Autodesk Fusion 360 part; units mm, degrees
note: some values were not read from the file. Chosen so that the rebuilt part matches the saved one: which face or edge a step refers to.
(part 2 of 2)
extrude "Extrusion14" cut sketch "Skizze12" against normal blind 11 contours L16 L18 L19 L481 L482 | L16 L475 L476 L477 | L18 L414 L418 | L16 L469 L470 L471 | L13 L408 L409 L410 L411 L412 L413 | L16 L463 L464 L465 | L16 L457 L458 L459 | L16 L451 L452 L453 | L14 L342 L343 L344 L345 L346 L347 | L16 L445 L446 L447 | L14 L276 L280 | L16 L439 L440 L441 | L14 L270 L271 L272 L273 L274 L275 | L16 L433 L434 L435 | L14 L204 L208 | L16 L427 L428 L429 | L14 L198 L199 L200 L201 L202 L203 | L16 L17 L20 L21 L422 L423 | L14 L132 L136 | L14 L15 L126 L127 L128 L129 L130 L131 | L17 L364 L365 | L15 L366 L367 L368 L369 L370 L371 | L15 L124 L125 | L15 L186 L187 L188 L189 L190 L191 | L15 L306 L307 L308 L309 L310 L311 | L15 L184 L185 | L15 L244 L245 | L15 L246 L247 L248 L249 L250 L251 | L24 L25 L26 L27 L28 L29 | L192 L193 L194 L195 L196 L197 | L252 L253 L254 L255 L256 L257 | L258 L259 L260 L261 L262 L263 | L264 L265 L266 L267 L268 L269 | L312 L313 L314 L315 L316 L317 | L318 L319 L320 L321 L322 L323 | L324 L325 L326 L327 L328 L329 | L330 L331 L332 L333 L334 L335 | L336 L337 L338 L339 L340 L341 | L372 L373 L374 L375 L376 L377 | L378 L379 L380 L381 L382 L383 | L384 L385 L386 L387 L388 L389 | L390 L391 L392 L393 L394 L395 | L396 L397 L398 L399 L400 L401 | L402 L403 L404 L405 L406 L407 bodies 1
chamfer "Fase2" distance 1 angle 45 6 edges at (152.6903, 75.2606, 26) (152.6903, 75.2606, 0) (162.0194, 75.2606, 1.4645) (163.4839, 75.2606, 13) (162.0194, 75.2606, 24.5355) (146.8968, 75.2606, 13) on bodies 1
copy_body "Körper->Berechn2" bodies 1 removing the originals makes body 2 in component "Rechter Halter"
sketch "Skizze13" plane through (0, 72.2606, 0) normal (0, -1, 0) x (1, 0, 0)
  arc A0 (158.4839, 0) -> (163.4839, 5) centre (158.4839, 5) ccw
  line L0 (163.4839, 5) -> (163.4839, 21)
  arc A1 (163.4839, 21) -> (158.4839, 26) centre (158.4839, 21) ccw
  line L1 (158.4839, 26) -> (149.4839, 26)
  line L2 (149.4839, 26) -> (149.4839, 0)
  line L3 (149.4839, 0) -> (158.4839, 0)
  circle A2 centre (158.4839, 22) radius 2
  circle A3 centre (158.4839, 4) radius 2
  line L4 (149.4839, 13) -> (163.4839, 13) construction
  line L5 (153.892, 8) -> (150.392, 8)
  line L6 (150.392, 8) -> (150.392, 18)
  line L7 (150.392, 18) -> (153.892, 18)
  line L8 (153.892, 18) -> (153.892, 8)
  line L9 (153.892, 8) -> (150.392, 18) construction
  line L10 (150.392, 8) -> (153.892, 18) construction
  point P0 (152.142, 13)
  dimension "d115" = 10
  dimension "d116" = 3.5
  constraint midpoint L2 L4.start
  constraint midpoint L0 L4.end
  constraint horizontal L5
  constraint perpendicular L5 L6
  constraint parallel L5 L7
  constraint parallel L6 L8
  constraint coincident L9 P0
  constraint coincident L10 P0
  constraint coincident L4 P0
  measures "d115" distance of L5.start L7.end
  measures "d116" distance of L6.end L7.end
extrude "Extrusion1" cut sketch "Skizze13" against normal blind 6 contours L5 L6 L7 L8 bodies 2 in component "Rechter Halter"
chamfer "Fase1'" distance 0.5 angle 45 3 edges at (153.892, 72.2606, 13) (152.142, 72.2606, 8) (152.142, 72.2606, 18) on bodies 2 in component "Rechter Halter"
chamfer "Fase2'" distance 0.5 angle 45 4 edges at (150.392, 75.2606, 13) (152.142, 75.2606, 18) (153.892, 75.2606, 13) (152.142, 75.2606, 8) on bodies 2 in component "Rechter Halter"
mirror "Komponente spiegeln1" about plane through (0, 0, 0) normal (0, 0, 1) of bodies 2 makes body 3 in component "Linker Halter"
split "Teilen1" by plane through (143.9247, 55.2606, 0) normal (-0.989138, 0.146987, 0) bodies 2 makes body 4 at (93.6088, 53.345, 0) in component "Rechter Halter"
move_body "Verschieben1" bodies 2 to x (1, 0, 0) y (0, 1, 0) z (0, 0, 1) at (0, 0, 3) in component "Rechter Halter"
extrude "Extrusion2" add 1 faces at (143.1322, 49.9272, 1) along direction (0.989138, -0.146987, 0) up to surface end surface through (149.4839, 72.2606, 3) normal (0.987975, -0.154616, 0) offset 0 on bodies 4 bodies 4 2 in component "Rechter Halter"
extrude "Extrusion3" add 1 faces at (144.869, 55.1203, 1) along direction (0.146987, 0.989138, 0) blind 6 on bodies 4 bodies 4 in component "Rechter Halter"
chamfer "Fase3" distance 3 angle 45 1 edges at (146.2231, 60.9849, 0) on bodies 4 in component "Rechter Halter"
delete_face "Fläche löschen1" 1 faces at (143.6596, 47.1233, 1) on bodies 4 in component "Rechter Halter"
mirror "Komponente spiegeln2" about plane through (0, 0, 0) normal (0, 0, 1) of bodies 4 makes body 5 in component "Linker Halter (1)"
copy_body "Körper->Berechn1" [suppressed] in component "Befestigung"
component "Rechter Halter" placed x (1, 0, 0) y (0, 1, 0) z (0, 0, 1) at (0, 0, 0)
component "Linker Halter (1)" placed x (-1, 0, 0) y (0, 1, 0) z (0, 0, -1) at (326.9678, 0, 0)
equation "d13 = d14"
named bodies: "Aufnahme", "Befestigung"
